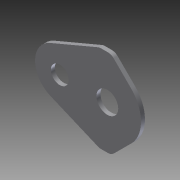
# Autodesk Inventor part: full plate
Saved by Autodesk Inventor 2012 (Build 160160000, 160)
## iProperties
Created: 2012-01-29
Part Number: full plate
Material: Default
Document SubType Name: Modeling
Designer: Antonella Wilby
Density: 1 g/cm^3
Author: Antonella Wilby
Autodesk Inventor part; units mm, degrees
ref_plane "YZ Plane" through (0, 0, 0) normal (1, 0, 0) x (0, 1, 0)
ref_plane "XZ Plane" through (0, 0, 0) normal (0, 1, 0) x (-1, 0, 0)
ref_plane "XY Plane" through (0, 0, 0) normal (0, 0, 1) x (1, 0, 0)
sketch "Sketch1" plane through (0, 0, 0) normal (0, 0, 1) x (1, 0, 0)
  line L0 (-149.86, 0) -> (87.9475, 0) projected
  line L1 (0, -137.1561) -> (0, 141.8112) projected
  line L2 (11.7901, -97.3036) -> (11.7901, 101.9587) construction
  circle A0 centre (0, 0) radius 50.8 construction
  circle A1 centre (0, 0) radius 17.4625
  line L3 (1.105, 69.85) -> (-10.1317, 69.85)
  line L4 (10.0665, 66.149) -> (38.0865, 38.2455)
  line L5 (-10.1317, -69.85) -> (1.105, -69.85)
  line L6 (10.0665, -66.149) -> (38.0865, -38.2455)
  arc A2 (38.0865, -38.2455) -> (38.0865, 38.2455) centre (0, 0) ccw
  circle A3 centre (-76.2, 0) radius 14.2875
  arc A4 (-91.6211, 36.5689) -> (-91.6211, -36.5689) centre (-76.2, 0) ccw
  line L7 (-15.0665, 68.8521) -> (-91.6211, 36.5689)
  line L8 (-15.0665, -68.8521) -> (-91.6211, -36.5689)
  line L9 (-63.5889, 6.715) -> (-63.5889, -6.715) construction
  arc A5 (-10.1317, 69.85) -> (-15.0665, 68.8521) centre (-10.1317, 57.15) ccw
  arc A6 (10.0665, 66.149) -> (1.105, 69.85) centre (1.105, 57.15) ccw
  arc A7 (1.105, -69.85) -> (10.0665, -66.149) centre (1.105, -57.15) ccw
  arc A8 (-15.0665, -68.8521) -> (-10.1317, -69.85) centre (-10.1317, -57.15) ccw
  point P0 (11.7901, -97.3036)
  point P1 (11.7901, 101.9587)
  point P2 (46.1798, 0)
  point P3 (6.35, 69.85)
  point P4 (-12.7, 69.85)
  point P5 (6.35, -69.85)
  dimension "d9" = 101.6
  dimension "d10" = 34.925
  dimension "d12" = 69.85
  dimension "d15" = 19.05
  dimension "d16" = 3.175
  dimension "d19" = 28.575
  dimension "d20" = 25.4
  dimension "d22" = 6.35
  dimension "d23" = 6.35
  dimension "d24" = 12.7
  dimension "d25" = 76.2
  constraints: 14 end point, 14 point on circle, 12 tangent, 9 centre point, 7 point on line, 3 coincident, 3 equal length, 3 equal radius, 2 concentric, 2 horizontal alignment, 2 perpendicular, 3 other
  measures "d9" diameter of A0
  measures "d10" diameter of A1
  measures "d12" distance from line of A2.centre L3
  measures "d15" distance of point (6.35, 69.85) point (-12.7, 69.85)
  measures "d16" radial gap between concentric circles of A2 A0
  measures "d19" diameter of A3
  measures "d20" radial gap between concentric circles of A4 A3
  measures "d22" distance from line of L1 point (6.35, 69.85)
  measures "d23" distance from line of L1 point (6.35, -69.85)
  measures "d24" radius of A5
  measures "d25" distance of point (0, 0) A3.centre
extrude "Extrusion1" add sketch "Sketch1" along normal mid plane 6.35 contours A4 L7 A5 L3 L1 A1 L0 A3 | L0 A3 A1 L1 L5 A8 L8 A4 | L1 L3 A6 L4 A2 L0 A1 | A1 L0 A2 L6 A7 L5 L1
body "Solid1"
